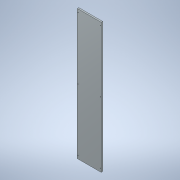
# Autodesk Inventor part: Back_plate_profile_V2
Saved by Autodesk Inventor 2022 (Build 260153000, 153)
## iProperties
Created: 2021-11-04
Part Number: Back_plate_profile_V2
Material: Generic
Document SubType Name: Modeling
Designer: espen
Density: 1 g/cm^3
Appearance: Zink
Author: espen
Autodesk Inventor part; units mm, degrees
ref_plane "YZ Plane" through (0, 0, 0) normal (1, 0, 0) x (0, 1, 0)
ref_plane "XZ Plane" through (0, 0, 0) normal (0, 1, 0) x (-1, 0, 0)
ref_plane "XY Plane" through (0, 0, 0) normal (0, 0, 1) x (1, 0, 0)
sketch "Sketch1" plane through (0, 0, 0) normal (0, 0, 1) x (1, 0, 0)
  line L0 (0, 0) -> (77, 0)
  line L1 (77, 0) -> (77, 420)
  line L2 (77, 420) -> (0, 420)
  line L3 (0, 420) -> (0, 0)
  line L4 (38.5, 420) -> (38.5, -89.9361)
  circle A0 centre (2.5, 410) radius 1
  circle A1 centre (2.5, 210) radius 1
  circle A2 centre (2.5, 10) radius 1
  circle A3 centre (74.5, 410) radius 1
  circle A4 centre (74.5, 210) radius 1
  circle A5 centre (74.5, 10) radius 1
  dimension "d0" = 420
  dimension "d1" = 77
  dimension "d2" = 2
  dimension "d3" = 2
  dimension "d4" = 2
  dimension "d5" = 2.5
  dimension "d6" = 10
  dimension "d7" = 2.5
  dimension "d8" = 210
  dimension "d9" = 2.5
  dimension "d10" = 410
  constraints: 10 end point, 6 centre point, 3 symmetric about line, 2 parallel, 1 horizontal, 1 midpoint, 1 perpendicular, 1 vertical, 3 other
  measures "d0" distance of L0.end L1.end
  measures "d1" distance of L0.start L0.end
  measures "d2" diameter of A0
  measures "d3" diameter of A1
  measures "d4" diameter of A2
  measures "d5" distance from line of L3 A0.centre
  measures "d6" distance from line of L2 A0.centre
  measures "d7" distance from line of L3 A1.centre
  measures "d8" distance from line of L2 A1.centre
  measures "d9" distance from line of L3 A2.centre
  measures "d10" distance from line of L2 A2.centre
extrude "Extrusion1" add sketch "Sketch1" along normal blind 5
body "Solid1"
